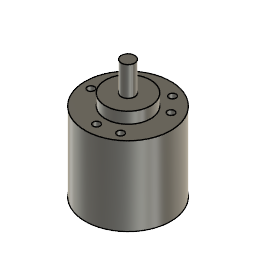
Encoder (Autodesk Fusion 360 design; units mm, degrees)
Autodesk Fusion 360 part; units mm, degrees
note: some values were not read from the file. Set by a fixed rule: which sketch regions a step uses.
sketch "Sketch1" plane through (0, 0, 0) normal (0, 0, 1) x (1, 0, 0)
  circle A0 centre (0, 0) radius 19
  dimension "d1" = 38
  constraint coincident A0.centre origin
  measures "d1" diameter of A0
extrude "Extrude1" add sketch "Sketch1" along normal blind 35
sketch "Sketch2" plane through (0, 0, 35) normal (0, 0, 1) x (-1, 0, 0)
  circle A0 centre (0, 0) radius 19
  circle A1 centre (0, 0) radius 10
  circle A2 centre (0, 0) radius 14 construction
  circle A3 centre (0, 0) radius 15 construction
  circle A4 centre (0, 14) radius 1.55
  line L0 (0, 0) -> (0, 1) construction
  line L1 (0, 1) -> (0, 14) construction
  line L2 (0, 0) -> (-8.8168, 12.1353) construction
  circle A5 centre (-8.8168, 12.1353) radius 1.55
  circle A6 centre (-12.1244, -7) radius 1.55
  circle A7 centre (12.1244, -7) radius 1.55
  circle A8 centre (-6.101, -13.7032) radius 1.55
  circle A9 centre (14.9178, 1.5679) radius 1.55
  dimension "d4" = 20
  dimension "d13" = 28
  dimension "d14" = 30
  dimension "d15" = 3.1
  dimension "d16" = 36
  dimension "d17" = 3.1
  dimension "d19" = 360
  dimension "d21" = 360
  constraint coincident A0.centre A1.centre
  constraint concentric A1 A3
  constraint coincident A2 A4.centre
  constraint vertical L0
  constraint coincident A4.centre L1.end
  constraint parallel L0 L1
  constraint coincident A3 L2.end
  constraint coincident L2.end A5.centre
  measures "d4" diameter of A1
  measures "d13" diameter of A2
  measures "d14" diameter of A3
  measures "d15" diameter of A4
  measures "d16" angle of L1 L2
  measures "d17" diameter of A5
extrude "Extrude2" add sketch "Sketch2" along normal blind 5 contours A1
sketch "Sketch3" plane through (0, 0, 40) normal (0, 0, 1) x (-1, 0, 0)
  circle A0 centre (0, 0) radius 10
  circle A1 centre (0, 0) radius 3
  line L0 (0, 3) -> (0, -2.58) construction
  line L1 (0, -2.58) -> (-1.5309, -2.58)
  line L2 (0, -2.58) -> (1.5309, -2.58)
  dimension "d7" = 6
  dimension "d8" = 5.58
  constraint coincident A0.centre A1.centre
  constraint coincident A1 L0.start
  constraint vertical L0
  constraint coincident A1 L1.end
  constraint perpendicular L0 L1
  constraint coincident A1 L2.end
  constraint perpendicular L0 L2
  measures "d7" diameter of A1
  measures "d8" distance of L0.start L0.end
extrude "Extrude3" add sketch "Sketch3" along normal blind 13 contours A1 L1 L2 picked at (0.0089, 1.1344)
extrude "Extrude4" add sketch "Sketch3" along normal blind 3 contours A1 L1 L2 picked at (0.1335, -2.8511)
extrude "Extrude5" cut sketch "Sketch2" against normal blind 6 contours A4 | A5 | A6 | A7 | A8 | A9
extrude "Extruir6" cut 1 faces at (-0.6852, 0.4836, 53) along direction (0, 0, -1) blind 10
extrude "Extruir7" cut 1 faces at (-0.782, -0.3761, 43) along direction (0, 0, -1) blind 5
extrude "Extruir8" add 1 faces at (-0.782, -0.3761, 38) along direction (0, 0, 1) blind 15
